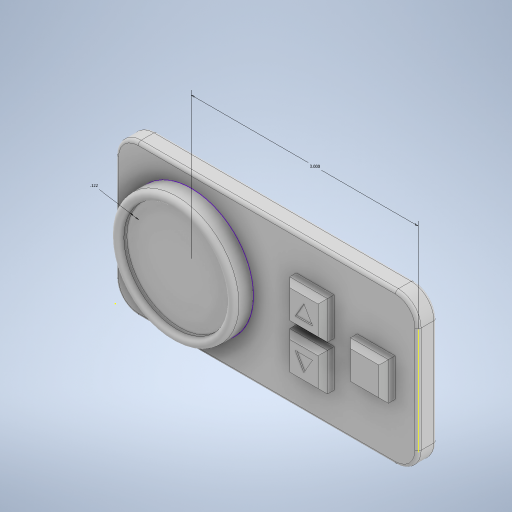
# Autodesk Inventor part: Control Panel
Saved by Autodesk Inventor 2023.2 (Build 272271030, 271C)
## iProperties
Created: 2023-02-27
Part Number: Control Panel
Material: Generic
Document SubType Name: Modeling
Designer: abhim
Density: 1 g/cm^3
Appearance: Default
Author: abhim
Autodesk Inventor part; units mm, degrees
ref_plane "YZ Plane" through (0, 0, 0) normal (1, 0, 0) x (0, 1, 0)
ref_plane "XZ Plane" through (0, 0, 0) normal (0, 1, 0) x (-1, 0, 0)
ref_plane "XY Plane" through (0, 0, 0) normal (0, 0, 1) x (1, 0, 0)
sketch "Sketch1" plane through (0, 0, 0) normal (0, 0, 1) x (1, 0, 0)
  line L0 (0, 0) -> (101.6, 0)
  line L1 (101.6, 0) -> (101.6, 50.8)
  line L2 (101.6, 50.8) -> (0, 50.8)
  line L3 (0, 50.8) -> (0, 0)
  dimension "d0" = 101.6
  dimension "d1" = 50.8
  constraints: 8 end point, 2 parallel, 1 horizontal, 1 perpendicular
  measures "d0" distance of L2.end L1.end
  measures "d1" distance of L1.end L0.end
extrude "Extrusion1" add sketch "Sketch1" along normal blind 6.35
fillet "Fillet1" radius 7.62 4 edges at (101.6, 50.8, 3.175) (101.6, 0, 3.175) (0, 50.8, 3.175) (0, 0, 3.175)
sketch "Sketch2" plane through (0, 0, 6.35) normal (0, 0, 1) x (1, 0, 0)
  circle A0 centre (25.4, 25.4) radius 20.8748
  line L0 (101.6, 7.62) -> (101.6, 43.18) projected
  circle A1 centre (25.4, 25.4) radius 17.78
  point P0 (0, 0)
  dimension "d5" = 76.2
  dimension "d13" = 3.0948
  constraints: 2 centre point, 1 coincident
  measures "d5" distance from line of L0 A0.centre
  measures "d13" radial gap between concentric circles of A0 A1
extrude "Extrusion2" add sketch "Sketch2" along normal blind 6.35 contours A0 | A1
extrude "Extrusion3" cut sketch "Sketch2" along normal blind 6.35 contours A1
extrude "Extrusion4" add sketch "Sketch2" along normal blind 3.81 contours A1
fillet "Fillet3" radius 1.5474 2 edges at (4.5252, 25.4, 12.7) (7.62, 25.4, 12.7)
sketch "Sketch3" plane through (0, 0, 6.35) normal (0, 0, 1) x (1, 0, 0)
  line L0 (60.7255, 39.2684) -> (73.4255, 39.2684)
  line L1 (73.4255, 39.2684) -> (73.4255, 26.5684)
  line L2 (73.4255, 26.5684) -> (60.7255, 26.5684)
  line L3 (60.7255, 26.5684) -> (60.7255, 39.2684)
  line L4 (60.7255, 11.5316) -> (73.4255, 11.5316)
  line L5 (73.4255, 11.5316) -> (73.4255, 24.2316)
  line L6 (73.4255, 24.2316) -> (60.7255, 24.2316)
  line L7 (60.7255, 24.2316) -> (60.7255, 11.5316)
  line L8 (93.98, 50.8) -> (7.62, 50.8) projected
  line L9 (7.62, 0) -> (93.98, 0) projected
  point P0 (0, 0)
  dimension "d15" = 12.7
  dimension "d16" = 12.7
  dimension "d17" = 12.7
  dimension "d18" = 12.7
  dimension "d19" = 11.5316
  dimension "d20" = 11.5316
  constraints: 16 end point, 4 parallel, 2 horizontal, 2 perpendicular
  measures "d15" distance of L1.end L2.end
  measures "d16" distance of L0.end L1.end
  measures "d17" distance of L6.end L5.end
  measures "d18" distance of L5.end L4.end
  measures "d19" distance between parallel lines of L8 L0
  measures "d20" distance between parallel lines of L9 L4
extrude "Extrusion5" add sketch "Sketch3" along normal blind 3.81
chamfer "Chamfer1" distance 1.5875 angle 45 4 edges at (67.0755, 39.2684, 10.16) (73.4255, 32.9184, 10.16) (67.0755, 26.5684, 10.16) (60.7255, 32.9184, 10.16)
chamfer "Chamfer2" distance 1.5875 angle 45 4 edges at (67.0755, 24.2316, 10.16) (60.7255, 17.8816, 10.16) (67.0755, 11.5316, 10.16) (73.4255, 17.8816, 10.16)
sketch "Sketch4" plane through (0, 0, 10.16) normal (0, 0, 1) x (1, 0, 0)
  line L0 (64.1926, 30.4165) -> (67.0755, 35.4098)
  line L1 (64.1926, 30.4165) -> (69.9584, 30.4165) construction
  line L2 (67.0755, 35.4098) -> (69.9584, 30.4165)
  line L3 (69.9584, 30.4165) -> (64.1926, 30.4165)
  line L4 (62.313, 28.1559) -> (62.313, 37.6809) projected
  line L5 (71.838, 37.6809) -> (71.838, 28.1559) projected
  line L6 (71.838, 28.1559) -> (62.313, 28.1559) projected
  line L7 (64.1926, 20.3835) -> (69.9584, 20.3835)
  line L8 (69.9584, 20.3835) -> (67.0755, 15.3902)
  line L9 (67.0755, 15.3902) -> (64.1926, 20.3835)
  line L10 (62.313, 22.6441) -> (71.838, 22.6441) projected
  line L11 (62.313, 13.1191) -> (62.313, 22.6441) projected
  point P0 (0, 0)
  dimension "d29" = 60
  dimension "d30" = 60
  dimension "d31" = 1.8796
  dimension "d33" = 5.7658
  dimension "d35" = 2.2606
  dimension "d36" = 4.9933
  dimension "d37" = 5.7658
  dimension "d38" = 5.7658
  dimension "d39" = 60
  dimension "d40" = 2.2606
  dimension "d41" = 1.8796
  constraints: 14 end point, 2 horizontal, 1 equal length, 1 perpendicular
  measures "d29" angle of L1 L0
  measures "d30" angle of L0 L2
  measures "d31" distance from line of L5 L1.end
  measures "d33" distance of L0.start L1.end
  measures "d35" distance between parallel lines of L6 L1
  measures "d36" distance from line of L0.end L1
  measures "d37" distance of L7.start L7.end
  measures "d38" distance of L7.end L8.end
  measures "d39" angle of L7 L8
  measures "d40" distance between parallel lines of L10 L7
  measures "d41" distance from line of L11 L7.start
extrude "Extrusion6" cut sketch "Sketch4" against normal blind 0.381
sketch "Sketch5" plane through (0, 0, 6.35) normal (0, 0, 1) x (1, 0, 0)
  line L0 (81.1657, 31.75) -> (93.8657, 31.75)
  line L1 (93.8657, 31.75) -> (93.8657, 19.05)
  line L2 (93.8657, 19.05) -> (81.1657, 19.05)
  line L3 (81.1657, 19.05) -> (81.1657, 31.75)
  line L4 (93.98, 50.8) -> (7.62, 50.8) projected
  line L5 (101.6, 7.62) -> (101.6, 43.18) projected
  point P0 (0, 0)
  dimension "d44" = 12.7
  dimension "d45" = 12.7
  dimension "d46" = 19.05
  dimension "d47" = 7.7343
  constraints: 8 end point, 2 parallel, 1 horizontal, 1 perpendicular
  measures "d44" distance of L1.end L2.end
  measures "d45" distance of L0.end L1.end
  measures "d46" distance between parallel lines of L4 L0
  measures "d47" distance between parallel lines of L5 L1
extrude "Extrusion7" add sketch "Sketch5" along normal blind 3.81
chamfer "Chamfer3" distance 1.5875 angle 45 4 edges at (87.5157, 31.75, 10.16) (93.8657, 25.4, 10.16) (87.5157, 19.05, 10.16) (81.1657, 25.4, 10.16)
fillet "Fillet4" radius 1.0316 8 edges at (2.2318, 48.5682, 6.35) (0, 25.4, 6.35) (2.2318, 2.2318, 6.35) (50.8, 0, 6.35) (99.3682, 2.2318, 6.35) (101.6, 25.4, 6.35) (99.3682, 48.5682, 6.35) (50.8, 50.8, 6.35)
fillet "Fillet5" radius 1.0316 8 edges at (2.2318, 48.5682, 0) (0, 25.4, 0) (2.2318, 2.2318, 0) (50.8, 0, 0) (99.3682, 2.2318, 0) (101.6, 25.4, 0) (99.3682, 48.5682, 0) (50.8, 50.8, 0)
body "Solid1"
